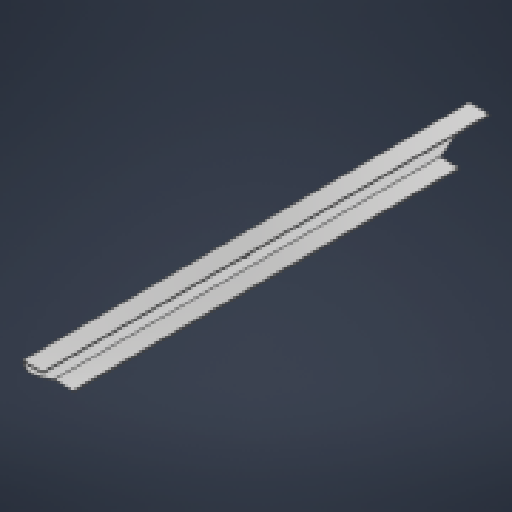
# Autodesk Inventor part: profile
Saved by Autodesk Inventor 2024 (Build 280153000, 153)
## iProperties
Created: 2024-04-30
Part Number: profile
Material: Aluminum 6061
Document SubType Name: Modeling
Designer: markm
Density: 2.7 g/cm^3
Appearance: Aluminum - Dark
Author: markm
Autodesk Inventor part; units mm, degrees
ref_plane "YZ Plane" through (0, 0, 0) normal (1, 0, 0) x (0, 1, 0)
ref_plane "XZ Plane" through (0, 0, 0) normal (0, 1, 0) x (-1, 0, 0)
ref_plane "XY Plane" through (0, 0, 0) normal (0, 0, 1) x (1, 0, 0)
sketch "Sketch1" plane through (0, 0, 0) normal (0, 0, 1) x (1, 0, 0)
  line L0 (-12.5, -20) -> (12.5, -20)
  line L1 (12.5, -20) -> (12.5, 20)
  line L2 (12.5, 20) -> (-12.5, 20)
  line L3 (-12.5, 20) -> (-12.5, -20)
  line L4 (-12.5, -20) -> (12.5, 20) construction
  line L5 (12.5, -20) -> (-12.5, 20) construction
  line L6 (-11, 18.5) -> (12.5, 18.5)
  line L7 (12.5, -18.5) -> (-11, -18.5)
  line L8 (-11, -18.5) -> (-11, 18.5)
  line L9 (0, 0) -> (-11, 0) construction
  dimension "d0" = 25
  dimension "d1" = 40
  dimension "d18" = 1.5
  dimension "d19" = 1.5
  constraints: 20 end point, 6 point on line, 4 parallel, 3 midpoint, 1 horizontal, 1 perpendicular, 1 other
  measures "d0" distance of L2.end L1.end
  measures "d1" distance of L1.end L0.end
  measures "d18" distance between parallel lines of L2 L6
  measures "d19" distance between parallel lines of L3 L8
extrude "Extrusion1" add sketch "Sketch1" along normal mid plane 550 contours L3 L2 L1 L6 L8 L7 L0
sketch "Sketch2" plane through (0, 0, 0) normal (1, 0, 0) x (0, 1, 0)
  line L0 (-20, -275) -> (-20, 275) projected
  line L1 (20, 275) -> (-20, 275) projected
  line L2 (20, -275) -> (20, 275) projected
  line L3 (-20, -275) -> (20, -275) projected
  line L4 (20, -275) -> (3.094, -275) construction
  line L5 (3.094, -275) -> (-20, -235) construction
  spline S0 degree 2 poles (20, -275) (3.094, -275) (-20, -235) knots 1 1 1 2 2 2
  point P0 (0, 0)
  dimension "d7" = 40
  dimension "d8" = 30
  constraints: 2 point on line, 3 other
  measures "d7" vertical distance of L4.end L5.end
  measures "d8" angle of L0 L5
extrude "Extrusion2" cut sketch "Sketch2" along normal through all both and the other way through all contours L0 S0 L3
mirror "Mirror1" about plane through (0, 0, 0) normal (0, 0, 1) of "Extrusion2"
sketch "Sketch3" plane through (-12.5, 20, -275) normal (-1, 0, 0) x (0, 0, 1)
  circle A0 centre (275, -20) radius 7
  line L0 (270, -24.899) -> (270, -15.101)
  line L1 (280, -15.101) -> (280, -24.899)
  circle A1 centre (275, -20) radius 12.5
  dimension "d11" = 14
  dimension "d12" = 10
  dimension "d26" = 25
  constraints: 4 end point, 4 point on circle, 2 centre point, 2 coincident, 2 parallel, 1 vertical
  measures "d11" diameter of A0
  measures "d12" distance between parallel lines of L1 L0
  measures "d26" diameter of A1
extrude "Extrusion3" cut sketch "Sketch3" against normal up to next contours A0 L1 | L1 A0 L0 | L0 A0
body "Solid1"
